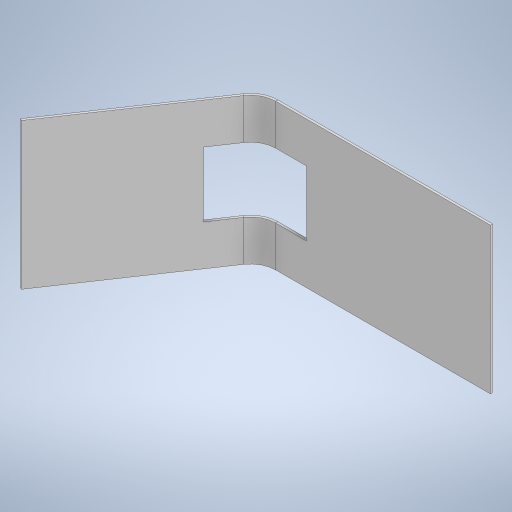
# Autodesk Inventor part: Ex 3
Saved by Autodesk Inventor 2023.2 (Build 272271000, 271)
## iProperties
Created: 2022-12-21
Part Number: Ex 3
Material: Generic
Document SubType Name: Sheet Metal
Designer: Felipe Coquito
Density: 1 g/cm^3
Sheet Metal Rule: Default_mm
Appearance: Default
Author: Felipe Coquito
Autodesk Inventor part; units mm, degrees
ref_plane "YZ Plane" through (0, 0, 0) normal (1, 0, 0) x (0, 1, 0)
ref_plane "XZ Plane" through (0, 0, 0) normal (0, 1, 0) x (-1, 0, 0)
ref_plane "XY Plane" through (0, 0, 0) normal (0, 0, 1) x (1, 0, 0)
sketch "Sketch1" plane through (0, 0, 0) normal (0, 0, 1) x (1, 0, 0)
  line L0 (-87.435, 31.905) -> (87.435, 31.905)
  line L1 (87.435, 31.905) -> (87.435, -31.905)
  line L2 (87.435, -31.905) -> (-87.435, -31.905)
  line L3 (-87.435, -31.905) -> (-87.435, 31.905)
  line L4 (-87.435, 31.905) -> (87.435, -31.905) construction
  line L5 (87.435, 31.905) -> (-87.435, -31.905) construction
  point P0 (0, 0)
  dimension "d0" = 174.87
  dimension "d1" = 63.81
  measures "d0" distance of L1.end L2.end
  measures "d1" distance of L0.end L1.end
extrude "Plate1" add sketch "Sketch1" along normal blind 1
sketch "Sketch2" plane through (0, 0, 1) normal (0, 0, 1) x (1, 0, 0)
  line L0 (-87.435, 31.905) -> (87.435, 31.905) projected
  line L1 (-11.865, 31.905) -> (-11.865, -31.905)
  line L2 (87.435, -31.905) -> (-87.435, -31.905) projected
  line L3 (-87.435, -31.905) -> (-87.435, 31.905) projected
  point P0 (0, 0)
  dimension "d3" = 75.57
  constraints: 2 end point, 2 point on line, 1 vertical
  measures "d3" distance between parallel lines of L1 L3
fold "Fold1" angle 56 bend radius 11 thickness 1 k factor 0.44 line from (-11.865, 31.905, 1) to (-11.865, -31.905, 1) line at bend centre moving side (-1, 0, 0) folds toward (0, 0, 1)
unfold all bends "Unfold1" k factor 0.44 fixed face at (56.1985, -10.635, 1)
sketch "Sketch3" plane through (-87.435, -31.905, 1) normal (0, 0, 1) x (1, 0, 0)
  line L0 (57.31, 46.05) -> (94.58, 46.05)
  line L1 (94.58, 46.05) -> (94.58, 17.76)
  line L2 (94.58, 17.76) -> (57.31, 17.76)
  line L3 (57.31, 17.76) -> (57.31, 46.05)
  line L4 (174.87, 63.81) -> (174.87, 0) projected
  point P0 (87.435, 31.905)
  dimension "d10" = 28.29
  dimension "d11" = 14.145
  dimension "d12" = 37.27
  dimension "d13" = 80.29
  constraints: 8 end point, 2 parallel, 1 horizontal, 1 perpendicular
  measures "d10" distance of L2.end L0.start
  measures "d11" vertical distance of L0.end point (87.435, 31.905)
  measures "d12" distance of L0.end L0.start
  measures "d13" distance from line of L4 L1.end
extrude "Cut1" cut sketch "Sketch3" against normal blind 1
refold all bends "Refold1"
equation "\"d2\" = Thickness"
equation "\"d4\" = BendReliefWidth"
equation "\"d5\" = BendReliefDepth"
equation "\"d6\" = MinimumRemnant"
equation "\"d7\" = TransitionRadius"
equation "\"d14\" = Thickness"
equation "\"BendRadius\" = Thickness"
equation "\"BendReliefWidth\" = Thickness"
equation "\"BendReliefDepth\" = 0.5 * Thickness"
equation "\"CornerReliefSize\" = 4 * Thickness"
equation "\"MinimumRemnant\" = 2 * Thickness"
equation "\"TransitionRadius\" = BendRadius"
equation "\"JacobiRadiusSize\" = BendRadius"
equation "\"GapSize\" = Thickness"
equation "\"Thickness\" = 1"
body "Solid1"
